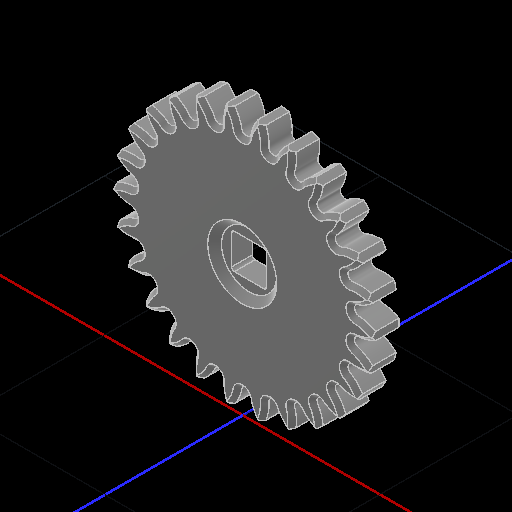
# Autodesk Inventor part: 26t_no_screwholes
Saved by Autodesk Inventor 2025.2 (Build 292293000, 293)
## iProperties
Created: 2025-11-16
Part Number: 26t_no_screwholes
Material: white pla
Document SubType Name: Modeling
Designer: cloudy
Density: 1 g/cm^3
Appearance: Smooth - Dark Gray
Author: cloudy
Autodesk Inventor part; units mm, degrees
ref_plane "YZ Plane" through (0, 0, 0) normal (1, 0, 0) x (0, 1, 0)
ref_plane "XZ Plane" through (0, 0, 0) normal (0, 1, 0) x (-1, 0, 0)
ref_plane "XY Plane" through (0, 0, 0) normal (0, 0, 1) x (1, 0, 0)
sketch "Sketch1" plane through (0, 0, 0) normal (0, 0, 1) x (1, 0, 0)
  spline S0 degree 3 poles (-2.1465, 23.7156) (-2.0953, 23.6384) (-1.9929, 23.4839) (-1.8471, 23.2472) (-1.7072, 23.0071) (-1.5742, 22.7629) (-1.4487, 22.5149) (-1.3314, 22.2629) (-1.223, 22.0069) (-1.1246, 21.7468) (-1.0388, 21.4825) (-0.9642, 21.2143) (-0.9273, 20.9855) (-0.8872, 20.8045) (-0.8448, 20.6721) (-0.7912, 20.5436) (-0.7206, 20.4236) (-0.6349, 20.3136) (-0.5472, 20.237) (-0.4701, 20.1855) (-0.4081, 20.1539) (-0.344, 20.1268) (-0.2768, 20.1086) (-0.2085, 20.0953) (-0.1158, 20.0903) (0, 20.0933) (0.1158, 20.0903) (0.2085, 20.0953) (0.2768, 20.1086) (0.344, 20.1268) (0.4081, 20.1539) (0.4701, 20.1855) (0.5472, 20.237) (0.6349, 20.3136) (0.7206, 20.4236) (0.7912, 20.5436) (0.8448, 20.6721) (0.8872, 20.8045) (0.9273, 20.9855) (0.9642, 21.2143) (1.0388, 21.4825) (1.1246, 21.7468) (1.223, 22.0069) (1.3314, 22.2629) (1.4487, 22.5149) (1.5742, 22.7629) (1.7072, 23.0071) (1.8471, 23.2472) (1.9929, 23.4839) (2.0953, 23.6384) (2.1465, 23.7156) knots 0 0 0 0 0.027794 0.055588 0.083382 0.111176 0.138969 0.166763 0.194556 0.222349 0.250141 0.277932 0.305721 0.319617 0.333508 0.347395 0.361282 0.375163 0.389047 0.395996 0.402941 0.409889 0.416835 0.423783 0.430729 0.444626 0.458524 0.465469 0.472418 0.479364 0.486312 0.493257 0.500206 0.514089 0.527971 0.541857 0.555745 0.569635 0.583532 0.611321 0.639112 0.666904 0.694696 0.72249 0.750283 0.778077 0.805871 0.833665 0.861459 0.889253 0.889253 0.889253 0.889253
  circle A0 centre (0, 0) radius 20.0921 construction
  circle A1 centre (0, 0) radius 20.8847 construction
  circle A2 centre (0, 0) radius 22.225 construction
  circle A3 centre (0, 0) radius 23.8125
  point P0 (-1.9942, 23.4831)
  point P1 (-1.848, 23.2467)
  point P2 (-1.7083, 23.0064)
  point P3 (-1.5755, 22.7623)
  point P4 (-1.4501, 22.5142)
  point P5 (-1.3329, 22.2622)
  point P6 (-1.2247, 22.0062)
  point P7 (-1.1267, 21.7461)
  point P8 (-1.0407, 21.4818)
  point P9 (-0.9693, 21.2133)
  point P10 (-0.9164, 20.9404)
  point P11 (-0.8852, 20.805)
  point P12 (-0.8429, 20.6727)
  point P13 (-0.7884, 20.545)
  point P14 (-0.7181, 20.4252)
  point P15 (-0.6317, 20.3166)
  point P16 (-0.5274, 20.225)
  point P17 (-0.4694, 20.1867)
  point P18 (-0.4077, 20.1547)
  point P19 (-0.3435, 20.1283)
  point P20 (-0.2766, 20.1094)
  point P21 (-0.2083, 20.0969)
  point P22 (-0.139, 20.0922)
  point P23 (0, 20.0921)
  point P24 (0.139, 20.0922)
  point P25 (0.2083, 20.0969)
  point P26 (0.2766, 20.1094)
  point P27 (0.3435, 20.1283)
  point P28 (0.4077, 20.1547)
  point P29 (0.4694, 20.1867)
  point P30 (0.5274, 20.225)
  point P31 (0.6317, 20.3166)
  point P32 (0.7181, 20.4252)
  point P33 (0.7884, 20.545)
  point P34 (0.8429, 20.6727)
  point P35 (0.8852, 20.805)
  point P36 (0.9164, 20.9404)
  point P37 (0.9693, 21.2133)
  point P38 (1.0407, 21.4818)
  point P39 (1.1267, 21.7461)
  point P40 (1.2247, 22.0062)
  point P41 (1.3329, 22.2622)
  point P42 (1.4501, 22.5142)
  point P43 (1.5755, 22.7623)
  point P44 (1.7083, 23.0064)
  point P45 (1.848, 23.2467)
  point P46 (1.9942, 23.4831)
  constraints: 4 centre point, 2 point on circle, 103 other
extrude "Extrusion1" add sketch "Sketch1" against normal blind 5.08
extrude "Extrusion2" cut sketch "Sketch1" against normal through all contours A3 S0 picked at (-0.2791, 22.7982)
chamfer "Chamfer1" distance 0.7937 angle 45 1 edges at (0, 20.0921, 0)
pattern_circular "Circular Pattern1" count 26 over 360 about axis through (0, 0, 0) along (0, 0, -1) of "Extrusion2", "Chamfer1"
sketch "Sketch2" plane through (0, 0, 0) normal (0, 0, 1) x (1, 0, 0)
  circle A0 centre (0, 0) radius 5.08
  dimension "d10" = 10.16
  constraints: 1 centre point, 1 coincident
  measures "d10" diameter of A0
extrude "Extrusion3" cut sketch "Sketch2" against normal blind 1.27
chamfer "Chamfer2" distance 1.27 angle 45 1 edges at (-5.08, 0, 0)
sketch "Sketch3" plane through (0, 0, -1.27) normal (0, 0, 1) x (1, 0, 0)
  line L0 (-3.2258, 3.2258) -> (3.2258, 3.2258)
  line L1 (3.2258, 3.2258) -> (3.2258, -3.2258)
  line L2 (3.2258, -3.2258) -> (-3.2258, -3.2258)
  line L3 (-3.2258, -3.2258) -> (-3.2258, 3.2258)
  line L4 (-3.2258, 3.2258) -> (3.2258, -3.2258) construction
  line L5 (3.2258, 3.2258) -> (-3.2258, -3.2258) construction
  point P0 (0, 0)
  dimension "d16" = 6.4516
  dimension "d17" = 6.4516
  constraints: 12 end point, 2 midpoint, 2 parallel, 1 horizontal, 1 perpendicular
  measures "d16" distance of L1.end L2.end
  measures "d17" distance of L0.end L1.end
extrude "Extrusion4" cut sketch "Sketch3" against normal through all
fillet "Fillet1" radius 0.508 4 edges at (-3.2258, 3.2258, -3.175) (-3.2258, -3.2258, -3.175) (3.2258, -3.2258, -3.175) (3.2258, 3.2258, -3.175)
equation "\"Module\" = 1.5875"
equation "\"PressureAngle\" = 20deg"
equation "\"UnitProfileClearance\" = 0.25"
equation "\"UnitRoundRadius\" = 0.35"
equation "\"HeadDiameter\" = 47.625"
equation "\"RootDiameter\" = 40.18419"
equation "\"BaseDiameter\" = 41.76934"
equation "\"PitchDiameter\" = 44.45"
equation "\"FaceWidth\" = 6.35"
equation "\"HelixAngle\" = 0"
equation "\"UnitCorrection\" = 0"
equation "\"UnitAddendumModification\" = 0"
equation "\"CircularPitch\" = 4.98728"
equation "\"UnitBacklashShift\" = -0.093562"
equation "\"TotalToolShift\" = -0.14853"
equation "\"IsInternal\" = 0"
body "Solid1"
